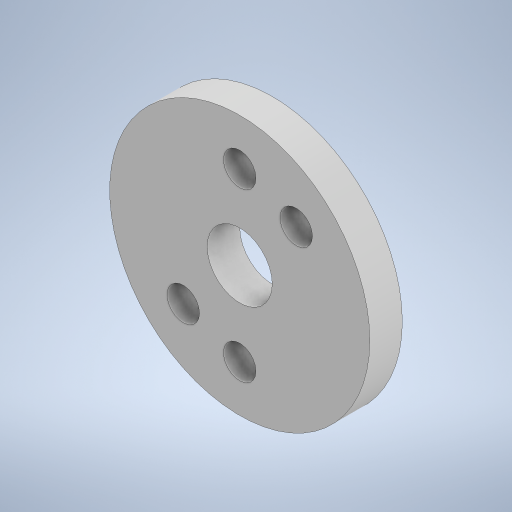
# Autodesk Inventor part: dondurgec
Saved by Autodesk Inventor 2023.2 (Build 272271000, 271)
## iProperties
Created: 2023-03-22
Part Number: dondurgec
Material: Generic
Document SubType Name: Modeling
Designer: sarp1
Density: 1 g/cm^3
Appearance: Default
Author: sarp1
Autodesk Inventor part; units mm, degrees
ref_plane "YZ Plane" through (0, 0, 0) normal (1, 0, 0) x (0, 1, 0)
ref_plane "XZ Plane" through (0, 0, 0) normal (0, 1, 0) x (-1, 0, 0)
ref_plane "XY Plane" through (0, 0, 0) normal (0, 0, 1) x (1, 0, 0)
sketch "Sketch1" plane through (0, 0, 0) normal (0, 0, 1) x (1, 0, 0)
  circle A0 centre (0, 0) radius 20
  circle A1 centre (0, 0) radius 5
  dimension "d0" = 40
  dimension "d1" = 10
  constraints: 2 centre point, 2 coincident
  measures "d0" diameter of A0
  measures "d1" diameter of A1
extrude "Extrusion1" add sketch "Sketch1" along normal blind 5
sketch "Sketch2" plane through (0, 0, 5) normal (0, 0, 1) x (1, 0, 0)
  circle A0 centre (0, 0) radius 5 projected
  line L0 (0, 0) -> (0, 12.85)
  circle A1 centre (0, 12.85) radius 2.5
  line L1 (0, 0) -> (8.6813, 9.474)
  circle A2 centre (8.6813, 9.474) radius 2.5
  circle A3 centre (0, 0) radius 20 projected
  line L2 (0, 0) -> (-20, 0)
  line L3 (0, 0) -> (20, 0) construction
  line L4 (0, 0) -> (-8.6813, -9.474)
  line L5 (0, 0) -> (12.85, 0) construction
  circle A4 centre (-8.6813, -9.474) radius 2.5
  line L6 (0, 0) -> (0, -12.85)
  circle A5 centre (0, -12.85) radius 2.5
  dimension "d4" = 12.85
  dimension "d5" = 5
  dimension "d6" = 12.85
  dimension "d8" = 5
  dimension "d15" = 90
  dimension "d17" = 47.5
  dimension "d18" = 42.5
  dimension "d20" = 12.85
  dimension "d21" = 132.5
  dimension "d22" = 5
  dimension "d23" = 12.85
  dimension "d24" = 5
  dimension "d25" = 42.5
  constraints: 14 end point, 4 centre point, 4 coincident, 3 horizontal, 1 equal length, 1 horizontal alignment, 1 perpendicular, 1 vertical, 1 other
  measures "d4" distance of L0.start L0.end
  measures "d5" diameter of A1
  measures "d6" distance of L0.start L1.end
  measures "d8" diameter of A2
  measures "d15" angle of L2 L0
  measures "d17" angle of L2 L1
  measures "d18" angle of L1 L0
  measures "d20" distance of L2.start L4.end
  measures "d21" angle of L4 L5
  measures "d22" diameter of A4
  measures "d23" distance of L2.start L6.end
  measures "d24" diameter of A5
  measures "d25" angle of L6 L4
extrude "Extrusion2" cut sketch "Sketch2" against normal blind 5 contours A5 | A4 | A1 | A2
body "Solid1"
